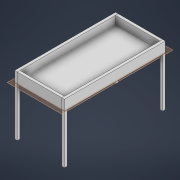
# Autodesk Inventor part: Mastersketch
Saved by Autodesk Inventor 2021 (Build 250183000, 183)
## iProperties
Created: 2021-11-16
Part Number: Mastersketch
Material: Generic
Document SubType Name: Modeling
Designer: jo_ki
Density: 1 g/cm^3
Appearance: Default
Author: jo_ki
Autodesk Inventor part; units mm, degrees
ref_plane "YZ Plane" through (0, 0, 0) normal (1, 0, 0) x (0, 1, 0)
ref_plane "XY Plane" through (0, 0, 0) normal (0, 0, 1) x (1, 0, 0)
sketch "Sketch3" plane through (0, 0, 0) normal (0, 1, 0) x (-1, 0, 0)
  line L0 (-360, 750) -> (360, 750)
  line L1 (360, 750) -> (360, -750)
  line L2 (360, -750) -> (-360, -750)
  line L3 (-360, -750) -> (-360, 750)
  line L4 (-360, 750) -> (360, -750) construction
  line L5 (360, 750) -> (-360, -750) construction
  line L6 (340, 770) -> (380, 770)
  line L7 (380, 770) -> (380, 730)
  line L8 (380, 730) -> (340, 730)
  line L9 (340, 730) -> (340, 770)
  line L10 (340, 770) -> (380, 730) construction
  line L11 (380, 770) -> (340, 730) construction
  line L12 (340, -730) -> (380, -730)
  line L13 (380, -730) -> (380, -770)
  line L14 (380, -770) -> (340, -770)
  line L15 (340, -770) -> (340, -730)
  line L16 (340, -730) -> (380, -770) construction
  line L17 (380, -730) -> (340, -770) construction
  line L18 (-380, -730) -> (-340, -730)
  line L19 (-340, -730) -> (-340, -770)
  line L20 (-340, -770) -> (-380, -770)
  line L21 (-380, -770) -> (-380, -730)
  line L22 (-380, -730) -> (-340, -770) construction
  line L23 (-340, -730) -> (-380, -770) construction
  line L24 (-380, 770) -> (-340, 770)
  line L25 (-340, 770) -> (-340, 730)
  line L26 (-340, 730) -> (-380, 730)
  line L27 (-380, 730) -> (-380, 770)
  line L28 (-380, 770) -> (-340, 730) construction
  line L29 (-340, 770) -> (-380, 730) construction
  point P0 (0, 0)
  dimension "d4" = 1500
  dimension "d5" = 720
  dimension "d6" = 40
  constraints: 60 end point, 10 midpoint, 10 parallel, 6 equal length, 5 horizontal, 5 perpendicular, 4 coincident, 1 point on line
  measures "d4" distance of L0.end L1.end
  measures "d5" distance of L0.start L0.end
  measures "d6" distance of L6.end L7.end
extrude "feetProfile" add sketch "Sketch3" along normal blind 746 contours L3 L26 L27 L24 L25 L0 | L0 L25 L26 L3 | L9 L6 L7 L8 L1 L0 | L0 L1 L8 L9 | L18 L19 L2 L3 | L3 L2 L19 L20 L21 L18 | L12 L13 L14 L15 L2 L1 | L1 L2 L15 L12
sketch "Sketch5" plane through (0, 0, 0) normal (0, 0, 1) x (1, 0, 0)
  line L0 (0, 1334.4) -> (0, -222.4) projected
  line L1 (340, 906) -> (380, 906)
  line L2 (380, 906) -> (380, 746)
  line L3 (380, 746) -> (340, 746)
  line L4 (340, 746) -> (340, 906)
  line L5 (340, 906) -> (380, 746) construction
  line L6 (380, 906) -> (340, 746) construction
  line L7 (-380, 906) -> (-340, 906)
  line L8 (-340, 906) -> (-340, 746)
  line L9 (-340, 746) -> (-380, 746)
  line L10 (-380, 746) -> (-380, 906)
  line L11 (-380, 906) -> (-340, 746) construction
  line L12 (-340, 906) -> (-380, 746) construction
  point P0 (0, 0)
  point P1 (360, 826)
  point P2 (-360, 826)
  dimension "d11" = 160
  dimension "d12" = 40
  dimension "d14" = 720
  dimension "d15" = 746
  constraints: 24 end point, 4 midpoint, 4 parallel, 2 horizontal, 2 perpendicular, 2 symmetric about line
  measures "d11" distance of L1.end L2.end
  measures "d12" distance of L2.end L3.end
  measures "d14" diameter of point (360, 826) L0
  measures "d15" distance from line of point (0, 0) L3
extrude "lengthProfileTall" add sketch "Sketch5" along normal mid plane 1540 separate body
sketch "Sketch6" plane through (0, 0, 0) normal (1, 0, 0) x (0, 1, 0)
  line L0 (906, 770) -> (746, 770)
  line L1 (746, 770) -> (746, 730)
  line L2 (746, 730) -> (906, 730)
  line L3 (906, 730) -> (906, 770)
  line L4 (906, 770) -> (746, 730) construction
  line L5 (746, 770) -> (906, 730) construction
  line L6 (906, -730) -> (746, -730)
  line L7 (746, -730) -> (746, -770)
  line L8 (746, -770) -> (906, -770)
  line L9 (906, -770) -> (906, -730)
  line L10 (906, -730) -> (746, -770) construction
  line L11 (746, -730) -> (906, -770) construction
  line L12 (-404, 0) -> (2424, 0) projected
  point P0 (0, 0)
  point P1 (826, 750)
  point P2 (826, -750)
  dimension "d22" = 160
  dimension "d23" = 1500
  dimension "d24" = 40
  dimension "d25" = 746
  constraints: 24 end point, 4 midpoint, 4 parallel, 2 horizontal, 2 perpendicular, 2 symmetric about line
  measures "d22" distance of L7.end L8.end
  measures "d23" distance of point (826, 750) point (826, -750)
  measures "d24" distance of L6.end L7.end
  measures "d25" distance from line of point (0, 0) L7
extrude "widthProfileTall" add sketch "Sketch6" along normal mid plane 680 separate body
sketch "Sketch7" plane through (0, 0, 0) normal (0, 1, 0) x (-1, 0, 0)
  line L0 (-360, 741) -> (360, 741)
  line L1 (360, 741) -> (360, -741)
  line L2 (360, -741) -> (-360, -741)
  line L3 (-360, -741) -> (-360, 741)
  line L4 (-360, 741) -> (360, -741) construction
  line L5 (360, 741) -> (-360, -741) construction
  point P0 (0, 0)
  dimension "d28" = 720
  dimension "d29" = 1482
  constraints: 12 end point, 2 midpoint, 2 parallel, 1 horizontal, 1 perpendicular
  measures "d28" distance of L1.end L2.end
  measures "d29" distance of L0.end L1.end
ref_plane "Work Plane1" through (0, 766, 0) normal (0, 1, 0) x (-1, 0, 0)
extrude "groundPlate" add sketch "Sketch7" along normal mid plane 8 from surface at 766 separate body
equation "\"d4\" = feet_lengthCenter"
equation "\"d5\" = feet_widthCenter"
equation "\"d6\" = profile_width"
equation "\"d7\" = feet_length"
equation "\"d11\" = profile_height"
equation "\"d12\" = profile_width"
equation "\"d14\" = feet_widthCenter"
equation "\"d15\" = feet_length"
equation "\"d16\" = feet_lengthCenter + profile_width"
equation "\"d22\" = profile_height"
equation "\"d23\" = feet_lengthCenter"
equation "\"d24\" = profile_width"
equation "\"d25\" = feet_length"
equation "\"d26\" = feet_widthCenter - profile_width"
equation "\"d28\" = groundPlate_width"
equation "\"d29\" = groundPlate_length"
equation "\"profile_width\" = 40"
equation "\"feet_widthCenter\" = 720"
equation "\"feet_lengthCenter\" = 1500"
equation "\"feet_length\" = 746"
equation "\"profile_height\" = 160"
equation "\"groundPlate_width\" = 720"
equation "\"groundPlate_length\" = 1482"
equation "\"d30\" = feet_length + 0.5 * profile_width"
body "Solid1"
body "Solid2"
body "Solid3"
body "Solid4"
